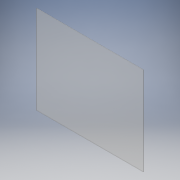
# Autodesk Inventor part: Plexi Sheet
Saved by Autodesk Inventor 2016 (Build 200138000, 138)
## iProperties
Created: 2016-11-17
Part Number: Plexi Sheet
Material: Polycarbonate, Clear
Document SubType Name: Modeling
Designer: 17kressc
Density: 1.2 g/cm^3
Appearance: Polycarbonate - Clear
Mass: 112.788 g
Surface Area: 1423.9 cm^2
Volume: 93.9901 cm^3
Author: 17kressc
Autodesk Inventor part; units mm, degrees
ref_plane "YZ Plane" through (0, 0, 0) normal (1, 0, 0) x (0, 1, 0)
ref_plane "XZ Plane" through (0, 0, 0) normal (0, 1, 0) x (-1, 0, 0)
ref_plane "XY Plane" through (0, 0, 0) normal (0, 0, 1) x (1, 0, 0)
sketch "Sketch1" plane through (0, 0, 0) normal (0, 0, 1) x (1, 0, 0)
  line L0 (0, 0) -> (292.1, 0)
  line L1 (292.1, 0) -> (292.1, 241.3)
  line L2 (292.1, 241.3) -> (0, 241.3)
  line L3 (0, 241.3) -> (0, 0)
  dimension "d0" = 292.1
  dimension "d1" = 241.3
  constraints: 8 end point, 2 parallel, 1 horizontal, 1 perpendicular
  measures "d0" distance of L2.end L1.end
  measures "d1" distance of L1.end L0.end
extrude "Extrusion1" add sketch "Sketch1" along normal blind 1.3335
body "Solid1"
